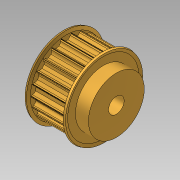
# Autodesk Inventor part: Engine Belt Wheel-1
Saved by Autodesk Inventor 2018.2 (Build 222227000, 227)
## iProperties
Created: 2019-08-01
Part Number: Engine Belt Wheel-1
Material: Generic
Document SubType Name: Modeling
Designer: NiveshandNisheeth
Density: 1 g/cm^3
Appearance: Brass - Satin
Author: NiveshandNisheeth
Autodesk Inventor part; units mm, degrees
ref_plane "YZ Plane" through (0, 0, 0) normal (1, 0, 0) x (0, 1, 0)
ref_plane "XZ Plane" through (0, 0, 0) normal (0, 1, 0) x (-1, 0, 0)
ref_plane "XY Plane" through (0, 0, 0) normal (0, 0, 1) x (1, 0, 0)
sketch "Sketch1" plane through (0, 0, 0) normal (1, 0, 0) x (0, 1, 0)
  line L0 (6, 0) -> (6, -40)
  line L1 (6, -40) -> (21.5, -40)
  line L2 (21.5, -40) -> (21.5, -30)
  line L3 (21.5, -30) -> (27.25, -30)
  line L4 (27.25, -30) -> (27.25, 0)
  line L5 (27.25, 0) -> (6, 0)
  line L6 (0, -48) -> (0, 8) projected
  point P0 (0, 0)
  dimension "d0" = 6
  dimension "d1" = 15.5
  dimension "d2" = 10
  dimension "d3" = 30
  dimension "d4" = 21.25
  constraints: 12 end point, 5 perpendicular, 1 horizontal alignment, 1 vertical
  measures "d0" distance from line of point (0, 0) L0
  measures "d1" distance of L0.end L1.end
  measures "d2" distance of L1.end L2.end
  measures "d3" distance of L3.end L4.end
  measures "d4" distance of L4.end L0.start
revolve "Revolution1" add sketch "Sketch1" angle 360 about axis through (0, 0, -10) along (0, 0, 1)
sketch "Sketch2" plane through (0, 0, 0) normal (0, 0, 1) x (1, 0, 0)
  arc A0 (-3, 26.5) -> (3, 26.5) centre (0, 26.5) ccw construction
  line L0 (-3.75, 28.5) -> (3.75, 28.5)
  line L1 (3.75, 28.5) -> (3.75, 26.5)
  line L2 (3.75, 26.5) -> (-3.75, 26.5) construction
  line L3 (-3.75, 26.5) -> (-3.75, 28.5)
  line L4 (-1.199, 23.75) -> (1.199, 23.75)
  line L5 (-3.75, 26.5) -> (-3.6742, 26.5)
  line L6 (3.6742, 26.5) -> (3.75, 26.5)
  arc A1 (-2.9394, 25.9) -> (-1.199, 23.75) centre (0, 26.5) ccw
  arc A2 (1.199, 23.75) -> (2.9394, 25.9) centre (0, 26.5) ccw
  arc A3 (-2.9394, 25.9) -> (-3.6742, 26.5) centre (-3.6742, 25.75) ccw
  arc A4 (3.6742, 26.5) -> (2.9394, 25.9) centre (3.6742, 25.75) ccw
  point P0 (0, 0)
  dimension "d6" = 3
  dimension "d7" = 2
  dimension "d8" = 7.5
  dimension "d9" = 26.5
  dimension "d10" = 2.75
  dimension "d11" = 0.75
  constraints: 14 end point, 14 point on circle, 5 centre point, 4 point on line, 4 tangent, 3 coincident, 3 equal length, 3 horizontal, 1 equal radius, 1 midpoint, 1 perpendicular, 1 vertical alignment
  measures "d6" radius of A0
  measures "d7" distance of L0.end L1.end
  measures "d8" distance of L0.start L0.end
  measures "d9" distance of point (0, 0) A0.centre
  measures "d10" distance from line of L4 A0.centre
  measures "d11" radius of A3
extrude "Extrusion1" cut sketch "Sketch2" against normal through all
pattern_circular "Circular Pattern1" count 22 over 360 about axis through (0, 0, -10) along (0, 0, 1) of "Extrusion1"
sketch "Sketch3" plane through (0, 0, 0) normal (1, 0, 0) x (0, 1, 0)
  line L0 (-23.75, -30) -> (-23.75, 0) construction
  line L1 (-23.75, 0) -> (-6, 0) construction
  line L2 (-6, 0) -> (-6, -40) construction
  line L3 (-6, -40) -> (-21.5, -40) construction
  line L4 (-21.5, -40) -> (-21.5, -30) construction
  line L5 (-21.5, -30) -> (-23.75, -30) construction
  line L6 (6, 0) -> (23.75, 0) construction
  line L7 (23.75, 0) -> (23.75, -30) construction
  line L8 (23.75, -30) -> (21.5, -30) construction
  line L9 (21.5, -30) -> (21.5, -40) construction
  line L10 (21.5, -40) -> (6, -40) construction
  line L11 (6, -40) -> (6, 0) construction
  line L12 (26.9907, 0) -> (26.9907, -30) construction
  line L13 (22.6907, 0) -> (27.6907, 0) construction
  line L14 (27.6907, 0) -> (27.6907, -1.5) construction
  line L15 (27.6907, -1.5) -> (22.6907, -1.5)
  line L16 (22.6907, -1.5) -> (22.6907, 0)
  line L17 (27.6907, -1.5) -> (27.3025, -0.0511) construction
  line L18 (27.3025, -0.0511) -> (29.7025, 0.592) construction
  line L19 (29.7025, 0.592) -> (30.0907, -0.8569)
  line L20 (30.0907, -0.8569) -> (27.6907, -1.5)
  line L21 (29.7025, 0.592) -> (27.4933, 0)
  line L22 (27.4933, 0) -> (22.6907, 0)
  line L23 (23.75, -15) -> (-23.75, -15)
  line L24 (-23.75, 0) -> (-23.75, -30) construction
  line L25 (27.6907, -28.5) -> (22.6907, -28.5)
  line L26 (22.6907, -28.5) -> (22.6907, -30)
  line L27 (29.7025, -30.592) -> (30.0907, -29.1431)
  line L28 (30.0907, -29.1431) -> (27.6907, -28.5)
  line L29 (29.7025, -30.592) -> (27.4933, -30)
  line L30 (27.4933, -30) -> (22.6907, -30)
  line L31 (0, -48.1184) -> (0, 8.7104) projected
  point P0 (0, 0)
  dimension "d17" = 0.7
  dimension "d18" = 5
  dimension "d19" = 1.5
  dimension "d20" = 2.4
  dimension "d21" = 165
  dimension "d22" = 1.5
  constraints: 34 end point, 6 symmetric about line, 4 parallel, 3 perpendicular, 3 point on line, 2 horizontal, 2 midpoint
  measures "d17" distance between parallel lines of L14 L12
  measures "d18" distance of L14.end L15.end
  measures "d19" distance of L15.end L13.start
  measures "d20" distance from line of L14 L19.end
  measures "d21" angle of L15 L20
  measures "d22" distance of L18.end L19.end
revolve "Revolution2" add sketch "Sketch3" angle 360 about axis through (0, 0, -10) along (0, 0, 1)
body "Solid1"
